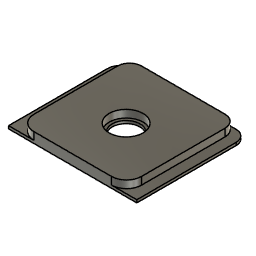
tapa1 (Autodesk Fusion 360 design; units mm, degrees)
Autodesk Fusion 360 part; units mm, degrees
sketch "Boceto2" plane through (0, 0, 0) normal (0, 0, 1) x (1, 0, 0)
  circle A0 centre (0, 0) radius 11.25
  circle A1 centre (0, 0) radius 9.25
  line L0 (-42.6, 38) -> (42.6, 38)
  line L1 (42.6, 38) -> (42.6, -39)
  line L2 (42.6, -39) -> (-42.6, -39)
  line L3 (-42.6, -39) -> (-42.6, 38)
  line L4 (-35.75, 38) -> (-35.75, -39)
  line L5 (35.75, 38) -> (35.75, -39)
  line L6 (35.75, -0.5) -> (42.6, -0.5)
  line L7 (-35.75, -0.5) -> (-42.6, -0.5)
  circle A2 centre (35.1, 30.5) radius 7.5
  circle A3 centre (-35.1, 30.5) radius 7.5
  line L8 (42.6, -35.5) -> (-42.6, -35.5)
  dimension "d1" = 22.5
  dimension "d3" = 2
  dimension "d4" = 39
  dimension "d5" = 77
  dimension "d6" = 85.2
  dimension "d7" = 42.6
  dimension "d14" = 71.5
  dimension "d15" = 15
  dimension "d16" = 3.5
  constraint coincident A0.centre A1.centre
  constraint horizontal L0
  constraint vertical L1
  constraint horizontal L2
  constraint vertical L3
  constraint coincident L0 L4.start
  constraint coincident L2 L4.end
  constraint perpendicular L2 L4
  constraint coincident L0 L5.start
  constraint coincident L2 L5.end
  constraint perpendicular L2 L5
  constraint midpoint L5 L6.start
  constraint midpoint L1 L6.end
  constraint midpoint L4 L7.start
  constraint midpoint L3 L7.end
  constraint equal L6 L7
  constraint tangent L0 A2
  constraint tangent L3 A3
  constraint tangent L0 A3
  constraint tangent L1 A2
  constraint horizontal A2.centre A3.centre
  constraint coincident L1 L8.start
  constraint coincident L3 L8.end
  constraint horizontal L8
  measures "d1" diameter of A0
  measures "d3" distance of A0 A1
  measures "d4" distance of A0.centre L2
  measures "d5" distance of L0.start L2.end
  measures "d6" distance of L0.start L0.end
  measures "d7" distance of A0.centre L3
  measures "d14" distance of L4 L5
  measures "d15" diameter of A2
  measures "d16" distance of L2 L8
extrude "Extruir1" add sketch "Boceto2" along normal blind 5 contours L0 L4 A3 | L0 L4 L5 A2 A3 L8 | L4 A3 | L0 L5 A2 | L5 A2 picked at (-32.8167, 30.5094) picked at (33.1671, 32.0923)
extrude "Extruir2" add sketch "Boceto2" against normal blind 1.8 contours A0 | L3 L4 L7 A3 | L4 A3 | L0 L4 L5 A2 A3 L8 | L4 A3 | L3 L4 L7 L8 | L5 A2 | L5 A2 | L1 L5 L6 A2 | L1 L5 L6 L8
fillet "Empalme1" radius 8 2 edges at (35.75, 38, 2.5) (-35.75, 38, 2.5)
fillet "Empalme2" radius 10 2 edges at (-35.75, -35.5, 2.5) (35.75, -35.5, 2.5)
equation "d7 = d6 / 2"
